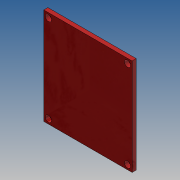
# Autodesk Inventor part: dimmer
Saved by Autodesk Inventor 2017 (Build 210142000, 142)
## iProperties
Part Number: dimmer
Material: Genérico
Document SubType Name: Modeling
Designer: FABLAB
Density: 1 g/cm^3
Appearance: Suave - Rojo
Author: FABLAB
Autodesk Inventor part; units mm, degrees
ref_plane "YZ Plane" through (0, 0, 0) normal (1, 0, 0) x (0, 1, 0)
ref_plane "XZ Plane" through (0, 0, 0) normal (0, 1, 0) x (-1, 0, 0)
ref_plane "XY Plane" through (0, 0, 0) normal (0, 0, 1) x (1, 0, 0)
sketch "Boceto1" plane through (0, 0, 0) normal (0, 1, 0) x (-1, 0, 0)
  line L0 (21.5, 23.5) -> (-21.5, 23.5)
  line L1 (-21.5, 23.5) -> (-21.5, -23.5)
  line L2 (-21.5, -23.5) -> (21.5, -23.5)
  line L3 (21.5, -23.5) -> (21.5, 23.5)
  line L4 (19.25, 21.25) -> (-19.25, 21.25) construction
  line L5 (-19.25, 21.25) -> (-19.25, -21.25) construction
  line L6 (-19.25, -21.25) -> (19.25, -21.25) construction
  line L7 (19.25, -21.25) -> (19.25, 21.25) construction
  circle A0 centre (19.25, 21.25) radius 1.5
  circle A1 centre (19.25, -21.25) radius 1.5
  circle A2 centre (-19.25, -21.25) radius 1.5
  circle A3 centre (-19.25, 21.25) radius 1.5
  point P0 (0, 0)
  point P1 (21.5, 0)
  point P2 (0, 23.5)
  dimension "d0" = 3
  dimension "d1" = 2.25
  dimension "d2" = 47
  dimension "d3" = 43
  dimension "d6" = 42.5
  dimension "d7" = 38.5
  constraints: 16 end point, 4 centre point, 4 parallel, 3 coincident, 3 equal radius, 2 midpoint, 2 perpendicular, 1 horizontal, 1 horizontal alignment, 1 vertical alignment, 3 other
  measures "d0" diameter of A0
  measures "d1" distance between parallel lines of L3 L7
  measures "d2" distance of L2.end L0.start
  measures "d3" distance of L0.start L0.end
  measures "d6" distance of L4.end L5.end
  measures "d7" distance of L4.start L4.end
extrude "Extrusión1" add sketch "Boceto1" along normal blind 2
